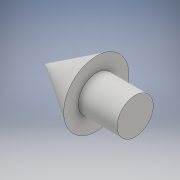
# Autodesk Inventor part: 探針
Saved by Autodesk Inventor 2017 (Build 210142000, 142)
## iProperties
Part Number: 探針
Material: 一般
Document SubType Name: Modeling
Designer: Brian
Density: 1 g/cm^3
Appearance: 預設
Author: Brian
Autodesk Inventor part; units mm, degrees
ref_plane "YZ Plane" through (0, 0, 0) normal (1, 0, 0) x (0, 1, 0)
ref_plane "XZ Plane" through (0, 0, 0) normal (0, 1, 0) x (-1, 0, 0)
ref_plane "XY Plane" through (0, 0, 0) normal (0, 0, 1) x (1, 0, 0)
sketch "草圖1" plane through (0, 0, 0) normal (0, 0, 1) x (1, 0, 0)
  line L0 (0, 0) -> (114.0317, 72.1786)
  line L1 (114.0317, 72.1786) -> (114.0317, 40)
  line L2 (114.0317, 40) -> (200, 40)
  line L3 (200, 40) -> (200, 0)
  line L4 (200, 0) -> (0, 0)
  dimension "d0" = 40
  dimension "d1" = 200
  constraints: 10 end point, 3 perpendicular, 1 vertical
  measures "d0" distance of L2.end L3.end
  measures "d1" distance of L3.end L0.start
revolve "迴轉1" add sketch "草圖1" angle 360 about axis through (200, 0, 0) along (-1, 0, 0)
